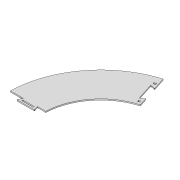
# Autodesk Inventor part: Level 2c - V2
Saved by Autodesk Inventor 2020 (Build 240168000, 168)
## iProperties
Created: 2020-07-30
Part Number: Level 2c - V2
Material: Generic
Document SubType Name: Modeling
Designer: Dan Wikman
Density: 1 g/cm^3
Appearance: Default
Author: Dan Wikman
Autodesk Inventor part; units mm, degrees
ref_plane "YZ Plane" through (0, 0, 0) normal (1, 0, 0) x (0, 1, 0)
ref_plane "XZ Plane" through (0, 0, 0) normal (0, 1, 0) x (-1, 0, 0)
ref_plane "XY Plane" through (0, 0, 0) normal (0, 0, 1) x (1, 0, 0)
sketch "Sketch1" plane through (0, 0, 0) normal (0, 1, 0) x (-1, 0, 0)
  line L0 (-545.8153, 185.3726) -> (-326.5965, 142.7608)
  line L1 (-545.8153, -185.3726) -> (-326.5965, -142.7608)
  arc A0 (-545.8153, -185.3726) -> (-545.8153, 185.3726) centre (0, 0) ccw
  arc A1 (374.3691, 3.75) -> (372.6191, 2) centre (374.3691, 2) ccw
  arc A2 (372.6191, -2) -> (374.3691, -3.75) centre (374.3691, -2) ccw
  line L2 (380.3691, 3.75) -> (374.3691, 3.75)
  line L3 (374.3691, -3.75) -> (380.3691, -3.75)
  line L4 (382.1191, 2) -> (382.1191, -2)
  arc A3 (380.3691, -3.75) -> (382.1191, -2) centre (380.3691, -2) ccw
  arc A4 (382.1191, 2) -> (380.3691, 3.75) centre (380.3691, 2) ccw
  line L5 (372.6191, -2) -> (372.6191, 2)
  line L6 (523.7076, 2) -> (523.7076, -2)
  arc A5 (523.7076, -2) -> (525.4576, -3.75) centre (525.4576, -2) ccw
  arc A6 (525.4576, 3.75) -> (523.7076, 2) centre (525.4576, 2) ccw
  line L7 (531.4576, -3.75) -> (525.4576, -3.75)
  line L8 (525.4576, 3.75) -> (531.4576, 3.75)
  arc A7 (531.4576, -3.75) -> (533.2076, -2) centre (531.4576, -2) ccw
  line L9 (533.2076, -2) -> (533.2076, 2)
  arc A8 (533.2076, 2) -> (531.4576, 3.75) centre (531.4576, 2) ccw
  arc A9 (-326.5965, -142.7608) -> (-326.5965, 142.7608) centre (0, 0) ccw
  line L10 (116.1792, 364.0349) -> (119.9834, 362.7989)
  arc A10 (121.107, 360.5937) -> (119.9834, 362.7989) centre (119.4426, 361.1345) ccw
  arc A11 (116.1792, 364.0349) -> (113.9741, 362.9114) centre (115.6384, 362.3706) ccw
  line L11 (119.2529, 354.8874) -> (121.107, 360.5937)
  line L12 (113.9741, 362.9114) -> (112.12, 357.205)
  line L13 (117.0478, 353.7638) -> (113.2435, 354.9999)
  arc A12 (112.12, 357.205) -> (113.2435, 354.9999) centre (113.7843, 356.6642) ccw
  arc A13 (117.0478, 353.7638) -> (119.2529, 354.8874) centre (117.5885, 355.4282) ccw
  arc A14 (163.7367, 497.4575) -> (165.9418, 498.5811) centre (164.2774, 499.1218) ccw
  arc A15 (158.8089, 500.8987) -> (159.9324, 498.6936) centre (160.4732, 500.3579) ccw
  line L14 (159.9324, 498.6936) -> (163.7367, 497.4575)
  line L15 (158.8089, 500.8987) -> (160.663, 506.605)
  line L16 (167.7959, 504.2874) -> (165.9418, 498.5811)
  arc A16 (162.8681, 507.7286) -> (160.663, 506.605) centre (162.3273, 506.0642) ccw
  line L17 (166.6723, 506.4925) -> (162.8681, 507.7286)
  arc A17 (167.7959, 504.2874) -> (166.6723, 506.4925) centre (166.1315, 504.8282) ccw
  line L18 (-310.3164, 222.986) -> (-307.9653, 226.222)
  arc A18 (-305.5209, 226.6092) -> (-307.9653, 226.222) centre (-306.5495, 225.1934) ccw
  arc A19 (-310.3164, 222.986) -> (-309.9293, 220.5416) centre (-308.9007, 221.9573) ccw
  line L19 (-300.6668, 223.0825) -> (-305.5209, 226.6092)
  line L20 (-309.9293, 220.5416) -> (-305.0752, 217.0148)
  line L21 (-300.2796, 220.6381) -> (-302.6308, 217.402)
  arc A20 (-305.0752, 217.0148) -> (-302.6308, 217.402) centre (-304.0466, 218.4306) ccw
  arc A21 (-300.2796, 220.6381) -> (-300.6668, 223.0825) centre (-301.6954, 221.6667) ccw
  arc A22 (-422.5128, 309.4456) -> (-422.8999, 311.89) centre (-423.9286, 310.4743) ccw
  arc A23 (-427.3083, 305.8224) -> (-424.8639, 306.2096) centre (-426.2797, 307.2382) ccw
  line L22 (-424.8639, 306.2096) -> (-422.5128, 309.4456)
  line L23 (-427.3083, 305.8224) -> (-432.1624, 309.3491)
  line L24 (-427.754, 315.4167) -> (-422.8999, 311.89)
  arc A24 (-432.5496, 311.7935) -> (-432.1624, 309.3491) centre (-431.1338, 310.7649) ccw
  line L25 (-430.1984, 315.0296) -> (-432.5496, 311.7935)
  arc A25 (-427.754, 315.4167) -> (-430.1984, 315.0296) centre (-428.7827, 314.001) ccw
  line L26 (-307.9653, -226.222) -> (-310.3164, -222.986)
  arc A26 (-309.9293, -220.5416) -> (-310.3164, -222.986) centre (-308.9007, -221.9573) ccw
  arc A27 (-307.9653, -226.222) -> (-305.5209, -226.6092) centre (-306.5495, -225.1934) ccw
  line L27 (-305.0752, -217.0148) -> (-309.9293, -220.5416)
  line L28 (-305.5209, -226.6092) -> (-300.6668, -223.0825)
  line L29 (-302.6308, -217.402) -> (-300.2796, -220.6381)
  arc A28 (-300.6668, -223.0825) -> (-300.2796, -220.6381) centre (-301.6954, -221.6667) ccw
  arc A29 (-302.6308, -217.402) -> (-305.0752, -217.0148) centre (-304.0466, -218.4306) ccw
  arc A30 (-424.8639, -306.2096) -> (-427.3083, -305.8224) centre (-426.2797, -307.2382) ccw
  arc A31 (-422.8999, -311.89) -> (-422.5128, -309.4456) centre (-423.9286, -310.4743) ccw
  line L30 (-422.5128, -309.4456) -> (-424.8639, -306.2096)
  line L31 (-422.8999, -311.89) -> (-427.754, -315.4167)
  line L32 (-432.1624, -309.3491) -> (-427.3083, -305.8224)
  arc A32 (-430.1984, -315.0296) -> (-427.754, -315.4167) centre (-428.7827, -314.001) ccw
  line L33 (-432.5496, -311.7935) -> (-430.1984, -315.0296)
  arc A33 (-432.1624, -309.3491) -> (-432.5496, -311.7935) centre (-431.1338, -310.7649) ccw
  line L34 (119.9834, -362.7989) -> (116.1792, -364.0349)
  arc A34 (113.9741, -362.9114) -> (116.1792, -364.0349) centre (115.6384, -362.3706) ccw
  arc A35 (119.9834, -362.7989) -> (121.107, -360.5937) centre (119.4426, -361.1345) ccw
  line L35 (112.12, -357.205) -> (113.9741, -362.9114)
  line L36 (121.107, -360.5937) -> (119.2529, -354.8874)
  line L37 (113.2435, -354.9999) -> (117.0478, -353.7638)
  arc A36 (119.2529, -354.8874) -> (117.0478, -353.7638) centre (117.5885, -355.4282) ccw
  arc A37 (113.2435, -354.9999) -> (112.12, -357.205) centre (113.7843, -356.6642) ccw
  arc A38 (159.9324, -498.6936) -> (158.8089, -500.8987) centre (160.4732, -500.3579) ccw
  arc A39 (165.9418, -498.5811) -> (163.7367, -497.4575) centre (164.2774, -499.1218) ccw
  line L38 (163.7367, -497.4575) -> (159.9324, -498.6936)
  line L39 (165.9418, -498.5811) -> (167.7959, -504.2874)
  line L40 (160.663, -506.605) -> (158.8089, -500.8987)
  arc A40 (166.6723, -506.4925) -> (167.7959, -504.2874) centre (166.1315, -504.8282) ccw
  line L41 (162.8681, -507.7286) -> (166.6723, -506.4925)
  arc A41 (160.663, -506.605) -> (162.8681, -507.7286) centre (162.3273, -506.0642) ccw
  line L42 (225.4462, 74.1184) -> (211.8442, 74.1184)
  line L43 (225.4462, 74.1184) -> (225.4462, 49.1184)
  arc A42 (405.4604, -13.75) -> (407.1248, -11.4592) centre (405.4604, -12) ccw
  arc A43 (496.0158, -11.1361) -> (497.5378, -13.75) centre (497.5378, -12) ccw
  line L44 (508.6578, 11.1361) -> (496.0158, -11.1361)
  arc A44 (508.6578, 11.1361) -> (507.1359, 13.75) centre (507.1359, 12) ccw
  arc A45 (416.8691, -2) -> (418.6191, -3.75) centre (418.6191, -2) ccw
  line L45 (399.6781, 11.4592) -> (407.1248, -11.4592)
  line L46 (416.8691, 2) -> (416.8691, -2)
  arc A46 (401.3425, 13.75) -> (399.6781, 11.4592) centre (401.3425, 12) ccw
  arc A47 (418.6191, 3.75) -> (416.8691, 2) centre (418.6191, 2) ccw
  line L47 (507.1359, 13.75) -> (401.3425, 13.75)
  line L48 (418.6191, -3.75) -> (487.1191, -3.75)
  line L49 (487.1191, 3.75) -> (418.6191, 3.75)
  arc A48 (487.1191, -3.75) -> (488.8691, -2.0136) centre (487.1326, -2.0136) ccw
  line L50 (488.8691, -2.0136) -> (488.8691, 2)
  arc A49 (488.8691, 2) -> (487.1191, 3.75) centre (487.1191, 2) ccw
  line L51 (405.4604, -13.75) -> (356.1697, -13.75)
  line L52 (497.5378, -13.75) -> (576.271, -13.75)
  arc A50 (163.8684, 468.2978) -> (166.8247, 468.9375) centre (165.1603, 469.4783) ccw
  line L53 (146.5928, 487.2036) -> (163.8684, 468.2978)
  arc A51 (146.5928, 487.2036) -> (143.6366, 486.5639) centre (145.3009, 486.0231) ccw
  line L54 (152.9839, 464.32) -> (149.1668, 465.5602)
  arc A52 (154.0946, 462.119) -> (152.9839, 464.32) centre (152.4473, 462.6685) ccw
  arc A53 (149.1668, 465.5602) -> (146.9616, 464.4366) centre (148.626, 463.8959) ccw
  arc A54 (110.9446, 385.9484) -> (112.609, 383.6576) centre (112.609, 385.4076) ccw
  arc A55 (138.3712, 381.3668) -> (136.7068, 383.6576) centre (136.7068, 381.9076) ccw
  line L55 (112.609, 383.6576) -> (136.7068, 383.6576)
  line L56 (126.9175, 397.0841) -> (130.7218, 395.8481)
  arc A56 (125.794, 399.2893) -> (126.9175, 397.0841) centre (127.4583, 398.7485) ccw
  line L57 (143.6366, 486.5639) -> (110.9446, 385.9484)
  line L58 (146.9616, 464.4366) -> (125.794, 399.2893)
  line L59 (132.9269, 396.9716) -> (154.0946, 462.119)
  arc A57 (130.7218, 395.8481) -> (132.9269, 396.9716) centre (131.2625, 397.5124) ccw
  line L60 (138.3712, 381.3668) -> (123.1395, 334.4885)
  line L61 (166.8247, 468.9375) -> (191.1546, 543.8173)
  line L62 (-394.3199, 288.9791) -> (-396.679, 285.732)
  arc A58 (-391.8835, 289.3553) -> (-394.3199, 288.9791) centre (-392.915, 287.9584) ccw
  arc A59 (-396.679, 285.732) -> (-396.2919, 283.2876) centre (-395.2632, 284.7034) ccw
  line L63 (-338.4298, 243.4115) -> (-336.0786, 246.6476)
  arc A60 (-340.8742, 243.0243) -> (-338.4298, 243.4115) centre (-339.8456, 244.4401) ccw
  line L64 (-396.2919, 283.2876) -> (-340.8742, 243.0243)
  line L65 (-336.4658, 249.092) -> (-391.8835, 289.3553)
  arc A61 (-336.0786, 246.6476) -> (-336.4658, 249.092) centre (-337.4944, 247.6762) ccw
  line L66 (-396.687, -285.7211) -> (-394.3279, -288.9681)
  arc A62 (-396.2919, -283.2876) -> (-396.687, -285.7211) centre (-395.2821, -284.7004) ccw
  arc A63 (-394.3279, -288.9681) -> (-391.8835, -289.3553) centre (-392.9121, -287.9395) ccw
  line L67 (-336.0786, -246.6476) -> (-338.4298, -243.4115)
  arc A64 (-336.4658, -249.092) -> (-336.0786, -246.6476) centre (-337.4944, -247.6762) ccw
  line L68 (-391.8835, -289.3553) -> (-336.4658, -249.092)
  line L69 (-340.8742, -243.0243) -> (-396.2919, -283.2876)
  arc A65 (-338.4298, -243.4115) -> (-340.8742, -243.0243) centre (-339.8456, -244.4401) ccw
  arc A66 (142.6862, -475.1804) -> (140.6706, -477.4355) centre (142.3349, -476.8947) ccw
  line L70 (167.775, -480.3211) -> (142.6862, -475.1804)
  arc A67 (167.775, -480.3211) -> (169.7906, -478.0659) centre (168.1263, -478.6067) ccw
  line L71 (149.1539, -465.5644) -> (152.971, -464.3241)
  arc A68 (146.9616, -464.4366) -> (149.1539, -465.5644) centre (148.6173, -463.9129) ccw
  arc A69 (152.971, -464.3241) -> (154.0946, -462.119) centre (152.4302, -462.6598) ccw
  arc A70 (137.0987, -377.4504) -> (134.4057, -376.5754) centre (135.4343, -377.9912) ccw
  arc A71 (112.2171, -389.8648) -> (114.9101, -390.7398) centre (113.8815, -389.324) ccw
  line L72 (134.4057, -376.5754) -> (114.9101, -390.7398)
  line L73 (130.7218, -395.8481) -> (126.9175, -397.0841)
  arc A72 (132.9269, -396.9716) -> (130.7218, -395.8481) centre (131.2625, -397.5124) ccw
  line L74 (169.7906, -478.0659) -> (137.0987, -377.4504)
  line L75 (154.0946, -462.119) -> (132.9269, -396.9716)
  line L76 (125.794, -399.2893) -> (146.9616, -464.4366)
  arc A73 (126.9175, -397.0841) -> (125.794, -399.2893) centre (127.4583, -398.7485) ccw
  line L77 (112.2171, -389.8648) -> (96.9855, -342.9865)
  line L78 (140.6706, -477.4355) -> (165.0005, -552.3153)
  line L79 (-432.5496, 311.7935) -> (-436.2232, 306.7372)
  line L80 (-435.8361, 304.2928) -> (-430.9801, 300.7647)
  line L81 (-428.5353, 301.1524) -> (-424.8639, 306.2096)
  arc A74 (-436.2232, 306.7372) -> (-435.8361, 304.2928) centre (-434.8075, 305.7085) ccw
  arc A75 (-430.9801, 300.7647) -> (-428.5353, 301.1524) centre (-429.9515, 302.1805) ccw
  line L82 (-310.3164, 222.986) -> (-313.9901, 217.9296)
  line L83 (-313.603, 215.4852) -> (-308.7469, 211.9571)
  line L84 (-306.3022, 212.3448) -> (-302.6308, 217.402)
  arc A76 (-313.9901, 217.9296) -> (-313.603, 215.4852) centre (-312.5743, 216.901) ccw
  arc A77 (-308.7469, 211.9571) -> (-306.3022, 212.3448) centre (-307.7183, 213.3729) ccw
  line L85 (-430.1984, -315.0296) -> (-426.5248, -320.086)
  arc A78 (-426.5248, -320.086) -> (-424.0804, -320.4731) centre (-425.109, -319.0573) ccw
  line L86 (-424.0804, -320.4731) -> (-419.2244, -316.945)
  arc A79 (-419.2244, -316.945) -> (-418.8376, -314.5001) centre (-420.253, -315.5292) ccw
  line L87 (-418.8376, -314.5001) -> (-422.5128, -309.4456)
  line L88 (-307.9653, -226.222) -> (-304.2917, -231.2784)
  arc A80 (-304.2917, -231.2784) -> (-301.8472, -231.6655) centre (-302.8759, -230.2498) ccw
  line L89 (-301.8472, -231.6655) -> (-296.9912, -228.1374)
  line L90 (-296.6045, -225.6925) -> (-300.2796, -220.6381)
  arc A81 (-296.9912, -228.1374) -> (-296.6045, -225.6925) centre (-298.0199, -226.7217) ccw
  line L91 (166.6723, -506.4925) -> (172.6164, -504.5612)
  arc A82 (172.6164, -504.5612) -> (173.74, -502.356) centre (172.0756, -502.8968) ccw
  line L92 (173.74, -502.356) -> (171.8852, -496.6475)
  arc A83 (171.8852, -496.6475) -> (169.6794, -495.5241) centre (170.2208, -497.1882) ccw
  line L93 (169.6794, -495.5241) -> (163.7367, -497.4575)
  line L94 (119.9834, -362.7989) -> (125.9275, -360.8675)
  arc A84 (125.9275, -360.8675) -> (127.0511, -358.6624) centre (125.3867, -359.2032) ccw
  line L95 (127.0511, -358.6624) -> (125.1963, -352.9538)
  line L96 (122.9905, -351.8304) -> (117.0478, -353.7638)
  arc A85 (125.1963, -352.9538) -> (122.9905, -351.8304) centre (123.5319, -353.4946) ccw
  line L97 (533.2076, 2) -> (533.2076, 8.25)
  arc A86 (533.2076, 8.25) -> (531.4576, 10) centre (531.4576, 8.25) ccw
  line L98 (531.4576, 10) -> (525.4552, 10)
  arc A87 (525.4552, 10) -> (523.7052, 8.2493) centre (525.4552, 8.25) ccw
  line L99 (523.7052, 8.2493) -> (523.7076, 2)
  line L100 (382.1191, 2) -> (382.1191, 8.25)
  arc A88 (382.1191, 8.25) -> (380.3691, 10) centre (380.3691, 8.25) ccw
  line L101 (380.3691, 10) -> (374.3668, 10)
  line L102 (372.6168, 8.2493) -> (372.6191, 2)
  arc A89 (374.3668, 10) -> (372.6168, 8.2493) centre (374.3668, 8.25) ccw
  line L103 (162.8681, 507.7286) -> (156.924, 509.6599)
  arc A90 (156.924, 509.6599) -> (154.7189, 508.5364) centre (156.3832, 507.9956) ccw
  line L104 (154.7189, 508.5364) -> (152.864, 502.8278)
  arc A91 (152.864, 502.8278) -> (153.9882, 500.6225) centre (154.5284, 502.287) ccw
  line L105 (153.9882, 500.6225) -> (159.9324, 498.6936)
  line L106 (116.1792, 364.0349) -> (110.2351, 365.9663)
  arc A92 (110.2351, 365.9663) -> (108.03, 364.8427) centre (109.6943, 364.3019) ccw
  line L107 (108.03, 364.8427) -> (106.1751, 359.1341)
  line L108 (107.2993, 356.9288) -> (113.2435, 354.9999)
  arc A93 (106.1751, 359.1341) -> (107.2993, 356.9288) centre (107.8395, 358.5934) ccw
  point P0 (494.5322, -13.75)
  point P1 (417.3817, -3.2374)
  point P2 (417.3817, 3.2374)
  point P3 (488.3566, 3.2374)
  point P4 (165.8959, 466.0791)
  point P5 (147.8315, 465.4551)
  point P6 (125.8991, 397.954)
  point P7 (132.057, 395.9532)
  point P8 (-396.9917, 284.4297)
  point P9 (-339.5718, 242.7117)
  point P10 (-335.766, 247.95)
  point P11 (-393.1859, -289.6679)
  point P12 (-335.766, -247.95)
  point P13 (-339.5718, -242.7117)
  point P14 (139.7418, -474.577)
  point P15 (153.9895, -463.4543)
  point P16 (132.057, -395.9532)
  point P17 (125.8991, -397.954)
  point P18 (-302.6308, 217.402)
  point P19 (113.2435, 354.9999)
  point P20 (372.6191, 2)
  point P21 (117.0478, -353.7638)
  dimension "d34" = 1152.87
  dimension "d45" = 7.5
  dimension "d48" = 712.87
  dimension "d60" = 360
  dimension "d62" = 13.602
  dimension "d63" = 25
  dimension "d72" = 7.5
  dimension "d74" = 3.5
  dimension "d75" = 3.5
  dimension "d79" = 0
  dimension "d80" = 8
  dimension "d81" = 1.75
  dimension "d84" = 8
  dimension "d85" = 1.75
  dimension "d88" = 360
  constraints: 218 end point, 205 point on circle, 94 centre point, 9 tangent, 6 point on line, 2 equal radius, 2 horizontal, 1 coincident, 1 vertical, 332 other
  measures "d34" diameter of A0
  measures "d45" distance between parallel lines of L2 L3
  measures "d48" diameter of A9
  measures "d62" distance of L42.start L42.end
  measures "d63" distance of L42.start L43.end
  measures "d72" distance between parallel lines of L49 L48
  measures "d74" diameter of A47
  measures "d75" diameter of A45
  measures "d79" angle of L23 L80
  measures "d80" distance from line of L25.end L80
  measures "d81" radius of A74
  measures "d84" distance from line of L82.start L83
  measures "d85" radius of A76
extrude "Extrusion1" add sketch "Sketch1" along normal blind 7 contours A0 L78 A66 L70 A67 L74 A70 L72 A71 L77 A9 L51 A42 L45 A46 L47 A44 L44 A43 L52
body "Solid1"
